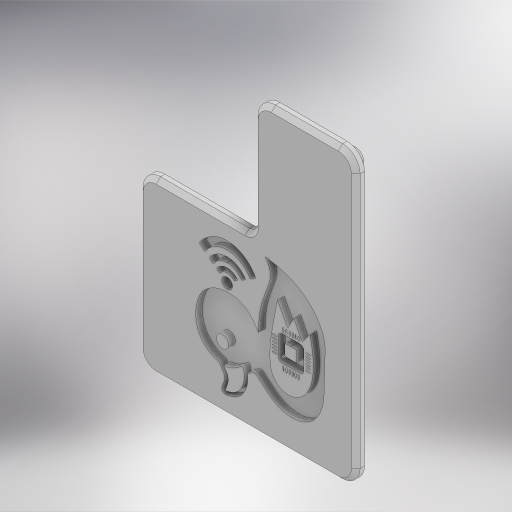
# Autodesk Inventor part: Case Top
Saved by Autodesk Inventor 2024 (Build 280153000, 153)
## iProperties
Created: 2024-10-30
Part Number: Case Top
Material: Generic
Document SubType Name: Modeling
Designer: Tejas
Mass: 8.4977 g
Surface Area: 64.1211 cm^2
Volume: 8.4977 cm^3
Density: 1 g/cm^3
Appearance: Default
Author: Tejas
Autodesk Inventor part; units mm, degrees
(part 1 of 2)
ref_plane "YZ Plane" through (0, 0, 0) normal (1, 0, 0) x (0, 1, 0)
ref_plane "XZ Plane" through (0, 0, 0) normal (0, 1, 0) x (-1, 0, 0)
ref_plane "XY Plane" through (0, 0, 0) normal (0, 0, 1) x (1, 0, 0)
sketch "Sketch1" plane through (0, 0, 0) normal (0, 0, 1) x (1, 0, 0)
  line L0 (-0.4879, 5.82) -> (-20.8921, 5.82) projected
  line L1 (-24.8921, 1.82) -> (-24.8921, -29.28) projected
  line L2 (-20.8921, -33.28) -> (20.8921, -33.28) projected
  line L3 (24.8921, -29.28) -> (24.8921, 29.28) projected
  line L4 (20.8921, 33.28) -> (5.5121, 33.28) projected
  line L5 (1.5121, 29.28) -> (1.5121, 7.82) projected
  line L6 (-22.8921, -29.28) -> (-22.8921, 1.82) projected
  line L7 (-20.8921, 3.82) -> (-0.4879, 3.82) projected
  line L8 (3.5121, 7.82) -> (3.5121, 29.28) projected
  line L9 (5.5121, 31.28) -> (20.8921, 31.28) projected
  line L10 (22.8921, 29.28) -> (22.8921, -29.28) projected
  line L11 (20.8921, -31.28) -> (-20.8921, -31.28) projected
  arc A0 (5.5121, 33.28) -> (1.5121, 29.28) centre (5.5121, 29.28) ccw projected
  arc A1 (-0.4879, 5.82) -> (1.5121, 7.82) centre (-0.4879, 7.82) ccw projected
  arc A2 (-20.8921, 5.82) -> (-24.8921, 1.82) centre (-20.8921, 1.82) ccw projected
  arc A3 (-24.8921, -29.28) -> (-20.8921, -33.28) centre (-20.8921, -29.28) ccw projected
  arc A4 (20.8921, -33.28) -> (24.8921, -29.28) centre (20.8921, -29.28) ccw projected
  arc A5 (24.8921, 29.28) -> (20.8921, 33.28) centre (20.8921, 29.28) ccw projected
  arc A6 (-0.4879, 3.82) -> (3.5121, 7.82) centre (-0.4879, 7.82) ccw projected
  arc A7 (5.5121, 31.28) -> (3.5121, 29.28) centre (5.5121, 29.28) ccw projected
  arc A8 (22.8921, 29.28) -> (20.8921, 31.28) centre (20.8921, 29.28) ccw projected
  arc A9 (20.8921, -31.28) -> (22.8921, -29.28) centre (20.8921, -29.28) ccw projected
  arc A10 (-22.8921, -29.28) -> (-20.8921, -31.28) centre (-20.8921, -29.28) ccw projected
  arc A11 (-20.8921, 3.82) -> (-22.8921, 1.82) centre (-20.8921, 1.82) ccw projected
  line L12 (22.6921, -29.28) -> (22.6921, 29.28)
  arc A12 (22.6921, 29.28) -> (20.8921, 31.08) centre (20.8921, 29.28) ccw
  line L13 (20.8921, 31.08) -> (5.5121, 31.08)
  arc A13 (5.5121, 31.08) -> (3.7121, 29.28) centre (5.5121, 29.28) ccw
  line L14 (3.7121, 29.28) -> (3.7121, 7.82)
  arc A14 (-0.4879, 3.62) -> (3.7121, 7.82) centre (-0.4879, 7.82) ccw
  line L15 (-0.4879, 3.62) -> (-20.8921, 3.62)
  arc A15 (-20.8921, 3.62) -> (-22.6921, 1.82) centre (-20.8921, 1.82) ccw
  line L16 (-22.6921, 1.82) -> (-22.6921, -29.28)
  arc A16 (-22.6921, -29.28) -> (-20.8921, -31.08) centre (-20.8921, -29.28) ccw
  line L17 (-20.8921, -31.08) -> (20.8921, -31.08)
  arc A17 (20.8921, -31.08) -> (22.6921, -29.28) centre (20.8921, -29.28) ccw
  point P0 (0, 0)
  dimension "d8" = 0.2
  constraints: 12 end point, 12 point on circle, 6 centre point, 11 other
  measures "d8" distance between parallel lines of L10 L12
extrude "Extrusion1" add sketch "Sketch1" against normal blind 2 contours A17 L17 A16 L16 A15 L15 A14 L14 A13 L13 A12 L12
sketch "Sketch2" plane through (0, 0, 0) normal (0, 0, 1) x (1, 0, 0)
  line L0 (-0.4879, 5.82) -> (-20.8921, 5.82) projected
  line L1 (-24.8921, 1.82) -> (-24.8921, -29.28) projected
  line L2 (-20.8921, -33.28) -> (20.8921, -33.28) projected
  line L3 (24.8921, -29.28) -> (24.8921, 29.28) projected
  line L4 (20.8921, 33.28) -> (5.5121, 33.28) projected
  line L5 (1.5121, 29.28) -> (1.5121, 7.82) projected
  line L6 (-22.8921, -29.28) -> (-22.8921, 1.82) projected
  line L7 (-20.8921, 3.82) -> (-0.4879, 3.82) projected
  line L8 (3.5121, 7.82) -> (3.5121, 29.28) projected
  line L9 (5.5121, 31.28) -> (20.8921, 31.28) projected
  line L10 (22.8921, 29.28) -> (22.8921, -29.28) projected
  line L11 (20.8921, -31.28) -> (-20.8921, -31.28) projected
  arc A0 (5.5121, 33.28) -> (1.5121, 29.28) centre (5.5121, 29.28) ccw projected
  arc A1 (-0.4879, 5.82) -> (1.5121, 7.82) centre (-0.4879, 7.82) ccw projected
  arc A2 (-20.8921, 5.82) -> (-24.8921, 1.82) centre (-20.8921, 1.82) ccw projected
  arc A3 (-24.8921, -29.28) -> (-20.8921, -33.28) centre (-20.8921, -29.28) ccw projected
  arc A4 (20.8921, -33.28) -> (24.8921, -29.28) centre (20.8921, -29.28) ccw projected
  arc A5 (24.8921, 29.28) -> (20.8921, 33.28) centre (20.8921, 29.28) ccw projected
  arc A6 (-0.4879, 3.82) -> (3.5121, 7.82) centre (-0.4879, 7.82) ccw projected
  arc A7 (5.5121, 31.28) -> (3.5121, 29.28) centre (5.5121, 29.28) ccw projected
  arc A8 (22.8921, 29.28) -> (20.8921, 31.28) centre (20.8921, 29.28) ccw projected
  arc A9 (20.8921, -31.28) -> (22.8921, -29.28) centre (20.8921, -29.28) ccw projected
  arc A10 (-22.8921, -29.28) -> (-20.8921, -31.28) centre (-20.8921, -29.28) ccw projected
  arc A11 (-20.8921, 3.82) -> (-22.8921, 1.82) centre (-20.8921, 1.82) ccw projected
  point P0 (0, 0)
extrude "Extrusion2" add sketch "Sketch2" along normal blind 2 contours A1 L5 A0 L4 A5 L3 A4 L2 A3 L1 A2 L0 | L6 A11 L7 A6 L8 A7 L9 A8 L10 A9 L11 A10
chamfer "Chamfer1" distance 1 angle 45 6 edges at (24.8921, 0, 2) (1.5121, 18.55, 2) (13.2021, 33.28, 2) (0, -33.28, 2) (-10.69, 5.82, 2) (-24.8921, -13.73, 2)
sketch "Sketch4" plane through (0, 0, 2) normal (0, 0, 1) x (1, 0, 0)
  spline S0 degree 3 poles (-4.7547, -28.9771) (-4.8805, -28.9733) (-5.0063, -28.9695) (-5.1321, -28.9657) (-5.8907, -28.5868) (-5.9479, -28.443) (-5.6662, -27.62) (-5.5577, -27.3029) (-5.4588, -26.9821) (-5.3379, -26.6697) (-5.0229, -25.8558) (-5.1151, -25.1226) (-5.6877, -24.4383) (-5.9033, -24.1806) (-6.0256, -23.8461) (-6.2014, -23.5532) (-6.2606, -23.4547) (-6.3372, -23.3352) (-6.4342, -23.2966) (-6.8229, -23.1422) (-7.2329, -23.0398) (-7.6166, -22.8751) (-9.6331, -22.0092) (-11.0259, -20.5743) (-11.5642, -18.4089) (-11.9734, -16.763) (-11.8527, -15.1208) (-11.3852, -13.5043) (-10.8906, -11.794) (-9.9099, -10.4354) (-8.3657, -9.5182) (-7.2061, -8.8296) (-5.9386, -8.5074) (-4.5948, -8.4534) (-3.1591, -8.3957) (-1.8032, -8.6617) (-0.5553, -9.3989) (0.7341, -10.1606) (1.5848, -11.3212) (2.3369, -12.5725) (2.4006, -12.6785) (2.4781, -12.7761) (2.5671, -12.9032) (2.5972, -12.8263) (2.6107, -12.8073) (2.6113, -12.7878) (2.6219, -12.4524) (2.6367, -12.1171) (2.6394, -11.7816) (2.6549, -9.9042) (2.9115, -8.0595) (3.4803, -6.2714) (3.8928, -4.9747) (4.3624, -3.6951) (4.8418, -2.4211) (5.558, -0.5179) (5.5086, 1.271) (4.1517, 2.8981) (4.2561, 2.8999) (4.364, 2.9203) (4.4642, 2.9007) (5.593, 2.6802) (6.7441, 2.5344) (7.8442, 2.2139) (11.5215, 1.1427) (14.5774, -0.8201) (16.5671, -4.1949) (17.399, -5.6059) (17.9137, -7.1329) (17.8745, -8.7927) (17.8045, -11.76) (17.7022, -14.7265) (17.6152, -17.6934) (17.5831, -18.7897) (17.4089, -19.8619) (17.0649, -20.9033) (16.6156, -22.2633) (15.9155, -23.4718) (14.7932, -24.3853) (12.9156, -25.9135) (10.761, -26.2581) (8.4518, -25.7287) (6.7621, -25.3413) (5.3811, -24.3687) (4.0943, -23.2515) (3.5164, -22.7497) (2.9519, -22.2318) (2.3622, -21.7443) (1.8553, -21.3253) (1.6817, -21.3258) (1.1206, -21.6528) (0.8489, -21.8111) (0.5904, -21.993) (0.3142, -22.1426) (0.1194, -22.2482) (0.0648, -22.3869) (0.078, -22.6006) (0.1026, -22.9968) (0.1327, -23.3977) (0.1005, -23.7917) (-0.0779, -25.9756) (-1.0908, -27.6067) (-3.1381, -28.4967) (-3.6499, -28.7191) (-4.2144, -28.8202) (-4.7547, -28.9771) knots 0 0 0 0 1 1 1 2 2 2 3 3 3 4 4 4 5 5 5 6 6 6 7 7 7 8 8 8 9 9 9 10 10 10 11 11 11 12 12 12 13 13 13 14 14 14 15 15 15 16 16 16 17 17 17 18 18 18 19 19 19 20 20 20 21 21 21 22 22 22 23 23 23 24 24 24 25 25 25 26 26 26 27 27 27 28 28 28 29 29 29 30 30 30 31 31 31 32 32 32 33 33 33 34 34 34 35 35 35 35
  line L0 (-4.7547, -28.9771) -> (-4.8805, -28.9733) construction
  line L1 (-4.8805, -28.9733) -> (-5.0063, -28.9695) construction
  line L2 (-5.0063, -28.9695) -> (-5.1321, -28.9657) construction
  line L3 (-5.1321, -28.9657) -> (-5.8907, -28.5868) construction
  line L4 (-5.8907, -28.5868) -> (-5.9479, -28.443) construction
  line L5 (-5.9479, -28.443) -> (-5.6662, -27.62) construction
  line L6 (-5.6662, -27.62) -> (-5.5577, -27.3029) construction
  line L7 (-5.5577, -27.3029) -> (-5.4588, -26.9821) construction
  line L8 (-5.4588, -26.9821) -> (-5.3379, -26.6697) construction
  line L9 (-5.3379, -26.6697) -> (-5.0229, -25.8558) construction
  line L10 (-5.0229, -25.8558) -> (-5.1151, -25.1226) construction
  line L11 (-5.1151, -25.1226) -> (-5.6877, -24.4383) construction
  line L12 (-5.6877, -24.4383) -> (-5.9033, -24.1806) construction
  line L13 (-5.9033, -24.1806) -> (-6.0256, -23.8461) construction
  line L14 (-6.0256, -23.8461) -> (-6.2014, -23.5532) construction
  line L15 (-6.2014, -23.5532) -> (-6.2606, -23.4547) construction
  line L16 (-6.2606, -23.4547) -> (-6.3372, -23.3352) construction
  line L17 (-6.3372, -23.3352) -> (-6.4342, -23.2966) construction
  line L18 (-6.4342, -23.2966) -> (-6.8229, -23.1422) construction
  line L19 (-6.8229, -23.1422) -> (-7.2329, -23.0398) construction
  line L20 (-7.2329, -23.0398) -> (-7.6166, -22.8751) construction
  line L21 (-7.6166, -22.8751) -> (-9.6331, -22.0092) construction
  line L22 (-9.6331, -22.0092) -> (-11.0259, -20.5743) construction
  line L23 (-11.0259, -20.5743) -> (-11.5642, -18.4089) construction
  line L24 (-11.5642, -18.4089) -> (-11.9734, -16.763) construction
  line L25 (-11.9734, -16.763) -> (-11.8527, -15.1208) construction
  line L26 (-11.8527, -15.1208) -> (-11.3852, -13.5043) construction
  line L27 (-11.3852, -13.5043) -> (-10.8906, -11.794) construction
  line L28 (-10.8906, -11.794) -> (-9.9099, -10.4354) construction
  line L29 (-9.9099, -10.4354) -> (-8.3657, -9.5182) construction
  line L30 (-8.3657, -9.5182) -> (-7.2061, -8.8296) construction
  line L31 (-7.2061, -8.8296) -> (-5.9386, -8.5074) construction
  line L32 (-5.9386, -8.5074) -> (-4.5948, -8.4534) construction
  line L33 (-4.5948, -8.4534) -> (-3.1591, -8.3957) construction
  line L34 (-3.1591, -8.3957) -> (-1.8032, -8.6617) construction
  line L35 (-1.8032, -8.6617) -> (-0.5553, -9.3989) construction
  line L36 (-0.5553, -9.3989) -> (0.7341, -10.1606) construction
  line L37 (0.7341, -10.1606) -> (1.5848, -11.3212) construction
  line L38 (1.5848, -11.3212) -> (2.3369, -12.5725) construction
  line L39 (2.3369, -12.5725) -> (2.4006, -12.6785) construction
  line L40 (2.4006, -12.6785) -> (2.4781, -12.7761) construction
  line L41 (2.4781, -12.7761) -> (2.5671, -12.9032) construction
  line L42 (2.5671, -12.9032) -> (2.5972, -12.8263) construction
  line L43 (2.5972, -12.8263) -> (2.6107, -12.8073) construction
  line L44 (2.6107, -12.8073) -> (2.6113, -12.7878) construction
  line L45 (2.6113, -12.7878) -> (2.6219, -12.4524) construction
  line L46 (2.6219, -12.4524) -> (2.6367, -12.1171) construction
  line L47 (2.6367, -12.1171) -> (2.6394, -11.7816) construction
  line L48 (2.6394, -11.7816) -> (2.6549, -9.9042) construction
  line L49 (2.6549, -9.9042) -> (2.9115, -8.0595) construction
  line L50 (2.9115, -8.0595) -> (3.4803, -6.2714) construction
  line L51 (3.4803, -6.2714) -> (3.8928, -4.9747) construction
  line L52 (3.8928, -4.9747) -> (4.3624, -3.6951) construction
  line L53 (4.3624, -3.6951) -> (4.8418, -2.4211) construction
  line L54 (4.8418, -2.4211) -> (5.558, -0.5179) construction
  line L55 (5.558, -0.5179) -> (5.5086, 1.271) construction
  line L56 (5.5086, 1.271) -> (4.1517, 2.8981) construction
  line L57 (4.1517, 2.8981) -> (4.2561, 2.8999) construction
  line L58 (4.2561, 2.8999) -> (4.364, 2.9203) construction
  line L59 (4.364, 2.9203) -> (4.4642, 2.9007) construction
  line L60 (4.4642, 2.9007) -> (5.593, 2.6802) construction
  line L61 (5.593, 2.6802) -> (6.7441, 2.5344) construction
  line L62 (6.7441, 2.5344) -> (7.8442, 2.2139) construction
  line L63 (7.8442, 2.2139) -> (11.5215, 1.1427) construction
  line L64 (11.5215, 1.1427) -> (14.5774, -0.8201) construction
  line L65 (14.5774, -0.8201) -> (16.5671, -4.1949) construction
  line L66 (16.5671, -4.1949) -> (17.399, -5.6059) construction
  line L67 (17.399, -5.6059) -> (17.9137, -7.1329) construction
  line L68 (17.9137, -7.1329) -> (17.8745, -8.7927) construction
  line L69 (17.8745, -8.7927) -> (17.8045, -11.76) construction
  line L70 (17.8045, -11.76) -> (17.7022, -14.7265) construction
  line L71 (17.7022, -14.7265) -> (17.6152, -17.6934) construction
  line L72 (17.6152, -17.6934) -> (17.5831, -18.7897) construction
  line L73 (17.5831, -18.7897) -> (17.4089, -19.8619) construction
  line L74 (17.4089, -19.8619) -> (17.0649, -20.9033) construction
  line L75 (17.0649, -20.9033) -> (16.6156, -22.2633) construction
  line L76 (16.6156, -22.2633) -> (15.9155, -23.4718) construction
  line L77 (15.9155, -23.4718) -> (14.7932, -24.3853) construction
  line L78 (14.7932, -24.3853) -> (12.9156, -25.9135) construction
  line L79 (12.9156, -25.9135) -> (10.761, -26.2581) construction
  line L80 (10.761, -26.2581) -> (8.4518, -25.7287) construction
  line L81 (8.4518, -25.7287) -> (6.7621, -25.3413) construction
  line L82 (6.7621, -25.3413) -> (5.3811, -24.3687) construction
  line L83 (5.3811, -24.3687) -> (4.0943, -23.2515) construction
  line L84 (4.0943, -23.2515) -> (3.5164, -22.7497) construction
  line L85 (3.5164, -22.7497) -> (2.9519, -22.2318) construction
  line L86 (2.9519, -22.2318) -> (2.3622, -21.7443) construction
  line L87 (2.3622, -21.7443) -> (1.8553, -21.3253) construction
  line L88 (1.8553, -21.3253) -> (1.6817, -21.3258) construction
  line L89 (1.6817, -21.3258) -> (1.1206, -21.6528) construction
  line L90 (1.1206, -21.6528) -> (0.8489, -21.8111) construction
  line L91 (0.8489, -21.8111) -> (0.5904, -21.993) construction
  line L92 (0.5904, -21.993) -> (0.3142, -22.1426) construction
  line L93 (0.3142, -22.1426) -> (0.1194, -22.2482) construction
  line L94 (0.1194, -22.2482) -> (0.0648, -22.3869) construction
  line L95 (0.0648, -22.3869) -> (0.078, -22.6006) construction
  line L96 (0.078, -22.6006) -> (0.1026, -22.9968) construction
  line L97 (0.1026, -22.9968) -> (0.1327, -23.3977) construction
  line L98 (0.1327, -23.3977) -> (0.1005, -23.7917) construction
  line L99 (0.1005, -23.7917) -> (-0.0779, -25.9756) construction
  line L100 (-0.0779, -25.9756) -> (-1.0908, -27.6067) construction
  line L101 (-1.0908, -27.6067) -> (-3.1381, -28.4967) construction
  line L102 (-3.1381, -28.4967) -> (-3.6499, -28.7191) construction
  line L103 (-3.6499, -28.7191) -> (-4.2144, -28.8202) construction
  line L104 (-4.2144, -28.8202) -> (-4.7547, -28.9771) construction
  spline S1 degree 3 poles (9.2856, -8.6579) (8.505, -7.185) (7.7646, -5.7881) (6.9636, -4.2766) (6.8805, -4.5615) (6.8204, -4.716) (6.7909, -4.8762) (6.3945, -7.025) (5.9735, -9.1697) (5.6179, -11.3252) (5.3014, -13.2442) (5.0982, -15.1784) (5.227, -17.1303) (5.2926, -18.1244) (5.4253, -19.0989) (6.0236, -19.9476) (6.7432, -20.9684) (7.6383, -21.725) (8.9273, -21.86) (10.737, -22.0495) (12.1366, -21.2461) (13.261, -19.925) (14.5002, -18.4692) (14.9367, -16.693) (15.102, -14.8381) (15.2756, -12.8887) (15.0995, -10.9567) (14.7416, -9.039) (14.6495, -8.5456) (14.5211, -8.059) (14.3809, -7.4445) (13.754, -8.2869) (13.2112, -9.0163) (12.6262, -9.8024) (12.2927, -9.142) (11.9917, -8.545) (11.6898, -7.9486) (11.3848, -7.3461) (11.0787, -6.7441) (10.7268, -6.0506) (10.2252, -6.9581) (9.7787, -7.7658) (9.2856, -8.6579) knots 0 0 0 0 1 1 1 2 2 2 3 3 3 4 4 4 5 5 5 6 6 6 7 7 7 8 8 8 9 9 9 10 10 10 11 11 11 12 12 12 13 13 13 14 14 14 14
  line L105 (9.2856, -8.6579) -> (8.505, -7.185) construction
  line L106 (8.505, -7.185) -> (7.7646, -5.7881) construction
  line L107 (7.7646, -5.7881) -> (6.9636, -4.2766) construction
  line L108 (6.9636, -4.2766) -> (6.8805, -4.5615) construction
  line L109 (6.8805, -4.5615) -> (6.8204, -4.716) construction
  line L110 (6.8204, -4.716) -> (6.7909, -4.8762) construction
  line L111 (6.7909, -4.8762) -> (6.3945, -7.025) construction
  line L112 (6.3945, -7.025) -> (5.9735, -9.1697) construction
  line L113 (5.9735, -9.1697) -> (5.6179, -11.3252) construction
  line L114 (5.6179, -11.3252) -> (5.3014, -13.2442) construction
  line L115 (5.3014, -13.2442) -> (5.0982, -15.1784) construction
  line L116 (5.0982, -15.1784) -> (5.227, -17.1303) construction
  line L117 (5.227, -17.1303) -> (5.2926, -18.1244) construction
  line L118 (5.2926, -18.1244) -> (5.4253, -19.0989) construction
  line L119 (5.4253, -19.0989) -> (6.0236, -19.9476) construction
  line L120 (6.0236, -19.9476) -> (6.7432, -20.9684) construction
  line L121 (6.7432, -20.9684) -> (7.6383, -21.725) construction
  line L122 (7.6383, -21.725) -> (8.9273, -21.86) construction
  line L123 (8.9273, -21.86) -> (10.737, -22.0495) construction
  line L124 (10.737, -22.0495) -> (12.1366, -21.2461) construction
  line L125 (12.1366, -21.2461) -> (13.261, -19.925) construction
  line L126 (13.261, -19.925) -> (14.5002, -18.4692) construction
  line L127 (14.5002, -18.4692) -> (14.9367, -16.693) construction
  line L128 (14.9367, -16.693) -> (15.102, -14.8381) construction
  line L129 (15.102, -14.8381) -> (15.2756, -12.8887) construction
  line L130 (15.2756, -12.8887) -> (15.0995, -10.9567) construction
  line L131 (15.0995, -10.9567) -> (14.7416, -9.039) construction
  line L132 (14.7416, -9.039) -> (14.6495, -8.5456) construction
  line L133 (14.6495, -8.5456) -> (14.5211, -8.059) construction
  line L134 (14.5211, -8.059) -> (14.3809, -7.4445) construction
  line L135 (14.3809, -7.4445) -> (13.754, -8.2869) construction
  line L136 (13.754, -8.2869) -> (13.2112, -9.0163) construction
  line L137 (13.2112, -9.0163) -> (12.6262, -9.8024) construction
  line L138 (12.6262, -9.8024) -> (12.2927, -9.142) construction
  line L139 (12.2927, -9.142) -> (11.9917, -8.545) construction
  line L140 (11.9917, -8.545) -> (11.6898, -7.9486) construction
  line L141 (11.6898, -7.9486) -> (11.3848, -7.3461) construction
  line L142 (11.3848, -7.3461) -> (11.0787, -6.7441) construction
  line L143 (11.0787, -6.7441) -> (10.7268, -6.0506) construction
  line L144 (10.7268, -6.0506) -> (10.2252, -6.9581) construction
  line L145 (10.2252, -6.9581) -> (9.7787, -7.7658) construction
  line L146 (9.7787, -7.7658) -> (9.2856, -8.6579) construction
  spline S2 degree 3 poles (-5.0153, -28.1685) (-4.8274, -28.1602) (-4.6842, -28.1705) (-4.5476, -28.1454) (-2.5666, -27.7822) (-1.1512, -26.3731) (-0.7618, -24.3571) (-0.5991, -23.5147) (-0.5871, -22.6719) (-0.8937, -21.8491) (-0.9953, -21.5764) (-1.1301, -21.4703) (-1.3993, -21.6813) (-1.6048, -21.8423) (-1.8351, -21.9712) (-2.0505, -22.12) (-2.978, -22.7607) (-3.9132, -23.3735) (-5.1093, -23.3633) (-5.3384, -23.3613) (-5.4382, -23.4962) (-5.2645, -23.7144) (-5.2059, -23.7881) (-5.1567, -23.8696) (-5.0954, -23.9408) (-4.3518, -24.8046) (-4.1806, -25.7695) (-4.5686, -26.8406) (-4.7209, -27.2611) (-4.8545, -27.6885) (-5.0153, -28.1685) knots 0 0 0 0 1 1 1 2 2 2 3 3 3 4 4 4 5 5 5 6 6 6 7 7 7 8 8 8 9 9 9 10 10 10 10
  line L147 (-5.0153, -28.1685) -> (-4.8274, -28.1602) construction
  line L148 (-4.8274, -28.1602) -> (-4.6842, -28.1705) construction
  line L149 (-4.6842, -28.1705) -> (-4.5476, -28.1454) construction
  line L150 (-4.5476, -28.1454) -> (-2.5666, -27.7822) construction
  line L151 (-2.5666, -27.7822) -> (-1.1512, -26.3731) construction
  line L152 (-1.1512, -26.3731) -> (-0.7618, -24.3571) construction
  line L153 (-0.7618, -24.3571) -> (-0.5991, -23.5147) construction
  line L154 (-0.5991, -23.5147) -> (-0.5871, -22.6719) construction
  line L155 (-0.5871, -22.6719) -> (-0.8937, -21.8491) construction
  line L156 (-0.8937, -21.8491) -> (-0.9953, -21.5764) construction
  line L157 (-0.9953, -21.5764) -> (-1.1301, -21.4703) construction
  line L158 (-1.1301, -21.4703) -> (-1.3993, -21.6813) construction
  line L159 (-1.3993, -21.6813) -> (-1.6048, -21.8423) construction
  line L160 (-1.6048, -21.8423) -> (-1.8351, -21.9712) construction
  line L161 (-1.8351, -21.9712) -> (-2.0505, -22.12) construction
  line L162 (-2.0505, -22.12) -> (-2.978, -22.7607) construction
  line L163 (-2.978, -22.7607) -> (-3.9132, -23.3735) construction
  line L164 (-3.9132, -23.3735) -> (-5.1093, -23.3633) construction
  line L165 (-5.1093, -23.3633) -> (-5.3384, -23.3613) construction
  line L166 (-5.3384, -23.3613) -> (-5.4382, -23.4962) construction
  line L167 (-5.4382, -23.4962) -> (-5.2645, -23.7144) construction
  line L168 (-5.2645, -23.7144) -> (-5.2059, -23.7881) construction
  line L169 (-5.2059, -23.7881) -> (-5.1567, -23.8696) construction
  line L170 (-5.1567, -23.8696) -> (-5.0954, -23.9408) construction
  line L171 (-5.0954, -23.9408) -> (-4.3518, -24.8046) construction
  line L172 (-4.3518, -24.8046) -> (-4.1806, -25.7695) construction
  line L173 (-4.1806, -25.7695) -> (-4.5686, -26.8406) construction
  line L174 (-4.5686, -26.8406) -> (-4.7209, -27.2611) construction
  line L175 (-4.7209, -27.2611) -> (-4.8545, -27.6885) construction
  line L176 (-4.8545, -27.6885) -> (-5.0153, -28.1685) construction
  spline S3 degree 3 poles (-7.051, -18.7799) (-7.0738, -19.5635) (-6.4782, -20.1949) (-5.6968, -20.2154) (-4.9245, -20.2357) (-4.2739, -19.6233) (-4.2516, -18.8549) (-4.2296, -18.0955) (-4.8598, -17.4325) (-5.6215, -17.4139) (-6.4023, -17.3948) (-7.028, -17.9928) (-7.051, -18.7799) knots 0 0 0 0 1 1 1 2 2 2 3 3 3 4 4 4 4
  line L177 (-7.051, -18.7799) -> (-7.0738, -19.5635) construction
  line L178 (-7.0738, -19.5635) -> (-6.4782, -20.1949) construction
  line L179 (-6.4782, -20.1949) -> (-5.6968, -20.2154) construction
  line L180 (-5.6968, -20.2154) -> (-4.9245, -20.2357) construction
  line L181 (-4.9245, -20.2357) -> (-4.2739, -19.6233) construction
  line L182 (-4.2739, -19.6233) -> (-4.2516, -18.8549) construction
  line L183 (-4.2516, -18.8549) -> (-4.2296, -18.0955) construction
  line L184 (-4.2296, -18.0955) -> (-4.8598, -17.4325) construction
  line L185 (-4.8598, -17.4325) -> (-5.6215, -17.4139) construction
  line L186 (-5.6215, -17.4139) -> (-6.4023, -17.3948) construction
  line L187 (-6.4023, -17.3948) -> (-7.028, -17.9928) construction
  line L188 (-7.028, -17.9928) -> (-7.051, -18.7799) construction
  spline S4 degree 3 poles (8.9341, -17.736) (8.9109, -17.6399) (8.8729, -17.5445) (8.8676, -17.4473) (8.857, -17.2539) (8.8547, -17.0587) (8.8704, -16.8659) (8.8751, -16.8074) (8.9423, -16.7183) (8.9946, -16.707) (9.0959, -16.6851) (9.1302, -16.7745) (9.1308, -16.8654) (9.1323, -17.0958) (9.1361, -17.3263) (9.1283, -17.5565) (9.1262, -17.617) (9.085, -17.6762) (9.0618, -17.736) (9.0192, -17.736) (8.9767, -17.736) (8.9341, -17.736) knots 0 0 0 0 1 1 1 2 2 2 3 3 3 4 4 4 5 5 5 6 6 6 7 7 7 7
  line L189 (8.9341, -17.736) -> (8.9109, -17.6399) construction
  line L190 (8.9109, -17.6399) -> (8.8729, -17.5445) construction
  line L191 (8.8729, -17.5445) -> (8.8676, -17.4473) construction
  line L192 (8.8676, -17.4473) -> (8.857, -17.2539) construction
  line L193 (8.857, -17.2539) -> (8.8547, -17.0587) construction
  line L194 (8.8547, -17.0587) -> (8.8704, -16.8659) construction
  line L195 (8.8704, -16.8659) -> (8.8751, -16.8074) construction
  line L196 (8.8751, -16.8074) -> (8.9423, -16.7183) construction
  line L197 (8.9423, -16.7183) -> (8.9946, -16.707) construction
  line L198 (8.9946, -16.707) -> (9.0959, -16.6851) construction
  line L199 (9.0959, -16.6851) -> (9.1302, -16.7745) construction
  line L200 (9.1302, -16.7745) -> (9.1308, -16.8654) construction
  line L201 (9.1308, -16.8654) -> (9.1323, -17.0958) construction
  line L202 (9.1323, -17.0958) -> (9.1361, -17.3263) construction
  line L203 (9.1361, -17.3263) -> (9.1283, -17.5565) construction
  line L204 (9.1283, -17.5565) -> (9.1262, -17.617) construction
  line L205 (9.1262, -17.617) -> (9.085, -17.6762) construction
  line L206 (9.085, -17.6762) -> (9.0618, -17.736) construction
  line L207 (9.0618, -17.736) -> (9.0192, -17.736) construction
  line L208 (9.0192, -17.736) -> (8.9767, -17.736) construction
  line L209 (8.9767, -17.736) -> (8.9341, -17.736) construction
  spline S5 degree 3 poles (5.7963, -14.2881) (5.8955, -14.2649) (5.9939, -14.2272) (6.0942, -14.2215) (6.2846, -14.2108) (6.4769, -14.2086) (6.6667, -14.2243) (6.7252, -14.2291) (6.7778, -14.3037) (6.8331, -14.3463) (6.781, -14.3927) (6.7311, -14.4758) (6.6763, -14.4791) (6.4377, -14.4938) (6.1974, -14.4894) (5.9581, -14.482) (5.9035, -14.4803) (5.8502, -14.4389) (5.7963, -14.4158) (5.7963, -14.3732) (5.7963, -14.3306) (5.7963, -14.2881) knots 0 0 0 0 1 1 1 2 2 2 3 3 3 4 4 4 5 5 5 6 6 6 7 7 7 7
  line L210 (5.7963, -14.2881) -> (5.8955, -14.2649) construction
  line L211 (5.8955, -14.2649) -> (5.9939, -14.2272) construction
  line L212 (5.9939, -14.2272) -> (6.0942, -14.2215) construction
  line L213 (6.0942, -14.2215) -> (6.2846, -14.2108) construction
  line L214 (6.2846, -14.2108) -> (6.4769, -14.2086) construction
  line L215 (6.4769, -14.2086) -> (6.6667, -14.2243) construction
  line L216 (6.6667, -14.2243) -> (6.7252, -14.2291) construction
  line L217 (6.7252, -14.2291) -> (6.7778, -14.3037) construction
  line L218 (6.7778, -14.3037) -> (6.8331, -14.3463) construction
  line L219 (6.8331, -14.3463) -> (6.781, -14.3927) construction
  line L220 (6.781, -14.3927) -> (6.7311, -14.4758) construction
  line L221 (6.7311, -14.4758) -> (6.6763, -14.4791) construction
  line L222 (6.6763, -14.4791) -> (6.4377, -14.4938) construction
  line L223 (6.4377, -14.4938) -> (6.1974, -14.4894) construction
  line L224 (6.1974, -14.4894) -> (5.9581, -14.482) construction
  line L225 (5.9581, -14.482) -> (5.9035, -14.4803) construction
  line L226 (5.9035, -14.4803) -> (5.8502, -14.4389) construction
  line L227 (5.8502, -14.4389) -> (5.7963, -14.4158) construction
  line L228 (5.7963, -14.4158) -> (5.7963, -14.3732) construction
  line L229 (5.7963, -14.3732) -> (5.7963, -14.3306) construction
  line L230 (5.7963, -14.3306) -> (5.7963, -14.2881) construction
  spline S6 degree 3 poles (5.7963, -11.5151) (5.9231, -11.4928) (6.0491, -11.4594) (6.1768, -11.4508) (6.3428, -11.4396) (6.5113, -11.4365) (6.6761, -11.4545) (6.7326, -11.4607) (6.7811, -11.541) (6.8332, -11.5874) (6.7805, -11.6291) (6.7296, -11.7038) (6.6748, -11.7069) (6.436, -11.7202) (6.196, -11.7169) (5.9567, -11.7096) (5.9026, -11.7079) (5.8497, -11.6661) (5.7963, -11.6428) (5.7963, -11.6003) (5.7963, -11.5577) (5.7963, -11.5151) knots 0 0 0 0 1 1 1 2 2 2 3 3 3 4 4 4 5 5 5 6 6 6 7 7 7 7
  line L231 (5.7963, -11.5151) -> (5.9231, -11.4928) construction
  line L232 (5.9231, -11.4928) -> (6.0491, -11.4594) construction
  line L233 (6.0491, -11.4594) -> (6.1768, -11.4508) construction
  line L234 (6.1768, -11.4508) -> (6.3428, -11.4396) construction
  line L235 (6.3428, -11.4396) -> (6.5113, -11.4365) construction
  line L236 (6.5113, -11.4365) -> (6.6761, -11.4545) construction
  line L237 (6.6761, -11.4545) -> (6.7326, -11.4607) construction
  line L238 (6.7326, -11.4607) -> (6.7811, -11.541) construction
  line L239 (6.7811, -11.541) -> (6.8332, -11.5874) construction
  line L240 (6.8332, -11.5874) -> (6.7805, -11.6291) construction
  line L241 (6.7805, -11.6291) -> (6.7296, -11.7038) construction
  line L242 (6.7296, -11.7038) -> (6.6748, -11.7069) construction
  line L243 (6.6748, -11.7069) -> (6.436, -11.7202) construction
  line L244 (6.436, -11.7202) -> (6.196, -11.7169) construction
  line L245 (6.196, -11.7169) -> (5.9567, -11.7096) construction
  line L246 (5.9567, -11.7096) -> (5.9026, -11.7079) construction
  line L247 (5.9026, -11.7079) -> (5.8497, -11.6661) construction
  line L248 (5.8497, -11.6661) -> (5.7963, -11.6428) construction
  line L249 (5.7963, -11.6428) -> (5.7963, -11.6003) construction
  line L250 (5.7963, -11.6003) -> (5.7963, -11.5577) construction
  line L251 (5.7963, -11.5577) -> (5.7963, -11.5151) construction
  spline S7 degree 3 poles (11.6888, -17.736) (11.6717, -17.4297) (11.6503, -17.1235) (11.6431, -16.817) (11.6422, -16.7787) (11.717, -16.7073) (11.7563, -16.7076) (11.801, -16.7079) (11.8824, -16.7699) (11.8839, -16.8078) (11.8949, -17.0771) (11.8918, -17.3472) (11.8869, -17.6169) (11.8862, -17.6569) (11.853, -17.6963) (11.8348, -17.736) (11.7861, -17.736) (11.7375, -17.736) (11.6888, -17.736) knots 0 0 0 0 1 1 1 2 2 2 3 3 3 4 4 4 5 5 5 6 6 6 6
  line L252 (11.6888, -17.736) -> (11.6717, -17.4297) construction
  line L253 (11.6717, -17.4297) -> (11.6503, -17.1235) construction
  line L254 (11.6503, -17.1235) -> (11.6431, -16.817) construction
  line L255 (11.6431, -16.817) -> (11.6422, -16.7787) construction
  line L256 (11.6422, -16.7787) -> (11.717, -16.7073) construction
  line L257 (11.717, -16.7073) -> (11.7563, -16.7076) construction
  line L258 (11.7563, -16.7076) -> (11.801, -16.7079) construction
  line L259 (11.801, -16.7079) -> (11.8824, -16.7699) construction
  line L260 (11.8824, -16.7699) -> (11.8839, -16.8078) construction
  line L261 (11.8839, -16.8078) -> (11.8949, -17.0771) construction
  line L262 (11.8949, -17.0771) -> (11.8918, -17.3472) construction
  line L263 (11.8918, -17.3472) -> (11.8869, -17.6169) construction
  line L264 (11.8869, -17.6169) -> (11.8862, -17.6569) construction
  line L265 (11.8862, -17.6569) -> (11.853, -17.6963) construction
  line L266 (11.853, -17.6963) -> (11.8348, -17.736) construction
  line L267 (11.8348, -17.736) -> (11.7861, -17.736) construction
  line L268 (11.7861, -17.736) -> (11.7375, -17.736) construction
  line L269 (11.7375, -17.736) -> (11.6888, -17.736) construction
  spline S8 degree 3 poles (5.7963, -12.9381) (5.8836, -12.9148) (5.9702, -12.8759) (6.0585, -12.8715) (6.261, -12.8615) (6.465, -12.8592) (6.6668, -12.8743) (6.725, -12.8787) (6.8139, -12.9452) (6.8255, -12.9972) (6.8482, -13.0996) (6.7571, -13.1329) (6.6677, -13.1338) (6.4375, -13.1361) (6.2071, -13.1394) (5.9771, -13.1315) (5.9162, -13.1295) (5.8565, -13.0888) (5.7963, -13.0658) (5.7963, -13.0232) (5.7963, -12.9807) (5.7963, -12.9381) knots 0 0 0 0 1 1 1 2 2 2 3 3 3 4 4 4 5 5 5 6 6 6 7 7 7 7
  line L270 (5.7963, -12.9381) -> (5.8836, -12.9148) construction
  line L271 (5.8836, -12.9148) -> (5.9702, -12.8759) construction
  line L272 (5.9702, -12.8759) -> (6.0585, -12.8715) construction
  line L273 (6.0585, -12.8715) -> (6.261, -12.8615) construction
  line L274 (6.261, -12.8615) -> (6.465, -12.8592) construction
  line L275 (6.465, -12.8592) -> (6.6668, -12.8743) construction
  line L276 (6.6668, -12.8743) -> (6.725, -12.8787) construction
  line L277 (6.725, -12.8787) -> (6.8139, -12.9452) construction
  line L278 (6.8139, -12.9452) -> (6.8255, -12.9972) construction
  line L279 (6.8255, -12.9972) -> (6.8482, -13.0996) construction
  line L280 (6.8482, -13.0996) -> (6.7571, -13.1329) construction
  line L281 (6.7571, -13.1329) -> (6.6677, -13.1338) construction
  line L282 (6.6677, -13.1338) -> (6.4375, -13.1361) construction
  line L283 (6.4375, -13.1361) -> (6.2071, -13.1394) construction
  line L284 (6.2071, -13.1394) -> (5.9771, -13.1315) construction
  line L285 (5.9771, -13.1315) -> (5.9162, -13.1295) construction
  line L286 (5.9162, -13.1295) -> (5.8565, -13.0888) construction
  line L287 (5.8565, -13.0888) -> (5.7963, -13.0658) construction
  line L288 (5.7963, -13.0658) -> (5.7963, -13.0232) construction
  line L289 (5.7963, -13.0232) -> (5.7963, -12.9807) construction
  line L290 (5.7963, -12.9807) -> (5.7963, -12.9381) construction
  spline S9 degree 3 poles (10.9956, -17.736) (10.9742, -17.5908) (10.9427, -17.4462) (10.9343, -17.3002) (10.925, -17.1376) (10.9285, -16.973) (10.9455, -16.8112) (10.9498, -16.77) (11.0284, -16.7055) (11.0696, -16.7079) (11.1128, -16.7104) (11.1857, -16.7791) (11.1875, -16.8213) (11.1986, -17.0813) (11.1956, -17.342) (11.1909, -17.6024) (11.1901, -17.6472) (11.1587, -17.6915) (11.1415, -17.736) (11.0929, -17.736) (11.0442, -17.736) (10.9956, -17.736) knots 0 0 0 0 1 1 1 2 2 2 3 3 3 4 4 4 5 5 5 6 6 6 7 7 7 7
  line L291 (10.9956, -17.736) -> (10.9742, -17.5908) construction
  line L292 (10.9742, -17.5908) -> (10.9427, -17.4462) construction
  line L293 (10.9427, -17.4462) -> (10.9343, -17.3002) construction
  line L294 (10.9343, -17.3002) -> (10.925, -17.1376) construction
  line L295 (10.925, -17.1376) -> (10.9285, -16.973) construction
  line L296 (10.9285, -16.973) -> (10.9455, -16.8112) construction
  line L297 (10.9455, -16.8112) -> (10.9498, -16.77) construction
  line L298 (10.9498, -16.77) -> (11.0284, -16.7055) construction
  line L299 (11.0284, -16.7055) -> (11.0696, -16.7079) construction
  line L300 (11.0696, -16.7079) -> (11.1128, -16.7104) construction
  line L301 (11.1128, -16.7104) -> (11.1857, -16.7791) construction
  line L302 (11.1857, -16.7791) -> (11.1875, -16.8213) construction
  line L303 (11.1875, -16.8213) -> (11.1986, -17.0813) construction
  line L304 (11.1986, -17.0813) -> (11.1956, -17.342) construction
  line L305 (11.1956, -17.342) -> (11.1909, -17.6024) construction
  line L306 (11.1909, -17.6024) -> (11.1901, -17.6472) construction
  line L307 (11.1901, -17.6472) -> (11.1587, -17.6915) construction
  line L308 (11.1587, -17.6915) -> (11.1415, -17.736) construction
  line L309 (11.1415, -17.736) -> (11.0929, -17.736) construction
  line L310 (11.0929, -17.736) -> (11.0442, -17.736) construction
  line L311 (11.0442, -17.736) -> (10.9956, -17.736) construction
  spline S10 degree 3 poles (9.6456, -17.736) (9.624, -17.609) (9.5903, -17.4827) (9.5836, -17.3549) (9.5742, -17.177) (9.5757, -16.9971) (9.5934, -16.8202) (9.5978, -16.7759) (9.6818, -16.7396) (9.7292, -16.6997) (9.7672, -16.7464) (9.8358, -16.7917) (9.838, -16.84) (9.8492, -17.0878) (9.8472, -17.3365) (9.8402, -17.5847) (9.8388, -17.6357) (9.7966, -17.6856) (9.7733, -17.736) (9.7307, -17.736) (9.6881, -17.736) (9.6456, -17.736) knots 0 0 0 0 1 1 1 2 2 2 3 3 3 4 4 4 5 5 5 6 6 6 7 7 7 7
  line L312 (9.6456, -17.736) -> (9.624, -17.609) construction
  line L313 (9.624, -17.609) -> (9.5903, -17.4827) construction
  line L314 (9.5903, -17.4827) -> (9.5836, -17.3549) construction
  line L315 (9.5836, -17.3549) -> (9.5742, -17.177) construction
  line L316 (9.5742, -17.177) -> (9.5757, -16.9971) construction
  line L317 (9.5757, -16.9971) -> (9.5934, -16.8202) construction
  line L318 (9.5934, -16.8202) -> (9.5978, -16.7759) construction
  line L319 (9.5978, -16.7759) -> (9.6818, -16.7396) construction
  line L320 (9.6818, -16.7396) -> (9.7292, -16.6997) construction
  line L321 (9.7292, -16.6997) -> (9.7672, -16.7464) construction
  line L322 (9.7672, -16.7464) -> (9.8358, -16.7917) construction
  line L323 (9.8358, -16.7917) -> (9.838, -16.84) construction
  line L324 (9.838, -16.84) -> (9.8492, -17.0878) construction
  line L325 (9.8492, -17.0878) -> (9.8472, -17.3365) construction
  line L326 (9.8472, -17.3365) -> (9.8402, -17.5847) construction
  line L327 (9.8402, -17.5847) -> (9.8388, -17.6357) construction
  line L328 (9.8388, -17.6357) -> (9.7966, -17.6856) construction
  line L329 (9.7966, -17.6856) -> (9.7733, -17.736) construction
  line L330 (9.7733, -17.736) -> (9.7307, -17.736) construction
  line L331 (9.7307, -17.736) -> (9.6881, -17.736) construction
  line L332 (9.6881, -17.736) -> (9.6456, -17.736) construction
  spline S11 degree 3 poles (14.4435, -11.6793) (14.1457, -11.6903) (13.8479, -11.7062) (13.55, -11.7067) (13.5084, -11.7067) (13.4322, -11.63) (13.4337, -11.5913) (13.4356, -11.5439) (13.5025, -11.4598) (13.5416, -11.4596) (13.8334, -11.4583) (14.1254, -11.4739) (14.4173, -11.4838) (14.426, -11.4841) (14.4348, -11.4805) (14.4435, -11.4786) (14.4435, -11.5455) (14.4435, -11.6124) (14.4435, -11.6793) knots 0 0 0 0 1 1 1 2 2 2 3 3 3 4 4 4 5 5 5 6 6 6 6
  line L333 (14.4435, -11.6793) -> (14.1457, -11.6903) construction
  line L334 (14.1457, -11.6903) -> (13.8479, -11.7062) construction
  line L335 (13.8479, -11.7062) -> (13.55, -11.7067) construction
  line L336 (13.55, -11.7067) -> (13.5084, -11.7067) construction
  line L337 (13.5084, -11.7067) -> (13.4322, -11.63) construction
  line L338 (13.4322, -11.63) -> (13.4337, -11.5913) construction
  line L339 (13.4337, -11.5913) -> (13.4356, -11.5439) construction
  line L340 (13.4356, -11.5439) -> (13.5025, -11.4598) construction
  line L341 (13.5025, -11.4598) -> (13.5416, -11.4596) construction
  line L342 (13.5416, -11.4596) -> (13.8334, -11.4583) construction
  line L343 (13.8334, -11.4583) -> (14.1254, -11.4739) construction
  line L344 (14.1254, -11.4739) -> (14.4173, -11.4838) construction
  line L345 (14.4173, -11.4838) -> (14.426, -11.4841) construction
  line L346 (14.426, -11.4841) -> (14.4348, -11.4805) construction
  line L347 (14.4348, -11.4805) -> (14.4435, -11.4786) construction
  line L348 (14.4435, -11.4786) -> (14.4435, -11.5455) construction
  line L349 (14.4435, -11.5455) -> (14.4435, -11.6124) construction
  line L350 (14.4435, -11.6124) -> (14.4435, -11.6793) construction
  spline S12 degree 3 poles (9.0983, -9.0888) (9.1093, -9.3716) (9.128, -9.6544) (9.125, -9.9371) (9.1244, -9.9945) (9.0499, -10.0891) (8.996, -10.0999) (8.8949, -10.1203) (8.8648, -10.0283) (8.8646, -9.9377) (8.8641, -9.7101) (8.8623, -9.4825) (8.866, -9.255) (8.8669, -9.1994) (8.8866, -9.1442) (8.8976, -9.0888) (8.9645, -9.0888) (9.0314, -9.0888) (9.0983, -9.0888) knots 0 0 0 0 1 1 1 2 2 2 3 3 3 4 4 4 5 5 5 6 6 6 6
  line L351 (9.0983, -9.0888) -> (9.1093, -9.3716) construction
  line L352 (9.1093, -9.3716) -> (9.128, -9.6544) construction
  line L353 (9.128, -9.6544) -> (9.125, -9.9371) construction
  line L354 (9.125, -9.9371) -> (9.1244, -9.9945) construction
  line L355 (9.1244, -9.9945) -> (9.0499, -10.0891) construction
  line L356 (9.0499, -10.0891) -> (8.996, -10.0999) construction
  line L357 (8.996, -10.0999) -> (8.8949, -10.1203) construction
  line L358 (8.8949, -10.1203) -> (8.8648, -10.0283) construction
  line L359 (8.8648, -10.0283) -> (8.8646, -9.9377) construction
  line L360 (8.8646, -9.9377) -> (8.8641, -9.7101) construction
  line L361 (8.8641, -9.7101) -> (8.8623, -9.4825) construction
  line L362 (8.8623, -9.4825) -> (8.866, -9.255) construction
  line L363 (8.866, -9.255) -> (8.8669, -9.1994) construction
  line L364 (8.8669, -9.1994) -> (8.8866, -9.1442) construction
  line L365 (8.8866, -9.1442) -> (8.8976, -9.0888) construction
  line L366 (8.8976, -9.0888) -> (8.9645, -9.0888) construction
  line L367 (8.9645, -9.0888) -> (9.0314, -9.0888) construction
  line L368 (9.0314, -9.0888) -> (9.0983, -9.0888) construction
  spline S13 degree 3 poles (14.4435, -14.4523) (14.1578, -14.4633) (13.872, -14.4815) (13.5863, -14.479) (13.5321, -14.4785) (13.4785, -14.396) (13.4247, -14.3513) (13.4785, -14.307) (13.5301, -14.2281) (13.5864, -14.2245) (13.819, -14.2101) (14.0531, -14.2165) (14.2866, -14.22) (14.339, -14.2207) (14.3912, -14.2405) (14.4435, -14.2516) (14.4435, -14.3185) (14.4435, -14.3854) (14.4435, -14.4523) knots 0 0 0 0 1 1 1 2 2 2 3 3 3 4 4 4 5 5 5 6 6 6 6
  line L369 (14.4435, -14.4523) -> (14.1578, -14.4633) construction
  line L370 (14.1578, -14.4633) -> (13.872, -14.4815) construction
  line L371 (13.872, -14.4815) -> (13.5863, -14.479) construction
  line L372 (13.5863, -14.479) -> (13.5321, -14.4785) construction
  line L373 (13.5321, -14.4785) -> (13.4785, -14.396) construction
  line L374 (13.4785, -14.396) -> (13.4247, -14.3513) construction
  line L375 (13.4247, -14.3513) -> (13.4785, -14.307) construction
  line L376 (13.4785, -14.307) -> (13.5301, -14.2281) construction
  line L377 (13.5301, -14.2281) -> (13.5864, -14.2245) construction
  line L378 (13.5864, -14.2245) -> (13.819, -14.2101) construction
  line L379 (13.819, -14.2101) -> (14.0531, -14.2165) construction
  line L380 (14.0531, -14.2165) -> (14.2866, -14.22) construction
  line L381 (14.2866, -14.22) -> (14.339, -14.2207) construction
  line L382 (14.339, -14.2207) -> (14.3912, -14.2405) construction
  line L383 (14.3912, -14.2405) -> (14.4435, -14.2516) construction
  line L384 (14.4435, -14.2516) -> (14.4435, -14.3185) construction
  line L385 (14.4435, -14.3185) -> (14.4435, -14.3854) construction
  line L386 (14.4435, -14.3854) -> (14.4435, -14.4523) construction
  spline S14 degree 3 poles (14.4435, -13.1023) (14.164, -13.1133) (13.8846, -13.1261) (13.605, -13.1343) (13.5144, -13.1369) (13.4274, -13.1133) (13.4269, -13.0001) (13.4264, -12.8854) (13.5121, -12.8683) (13.6043, -12.8683) (13.8256, -12.8684) (14.047, -12.8661) (14.2683, -12.8699) (14.3269, -12.8709) (14.3851, -12.8905) (14.4435, -12.9016) (14.4435, -12.9685) (14.4435, -13.0354) (14.4435, -13.1023) knots 0 0 0 0 1 1 1 2 2 2 3 3 3 4 4 4 5 5 5 6 6 6 6
  line L387 (14.4435, -13.1023) -> (14.164, -13.1133) construction
  line L388 (14.164, -13.1133) -> (13.8846, -13.1261) construction
  line L389 (13.8846, -13.1261) -> (13.605, -13.1343) construction
  line L390 (13.605, -13.1343) -> (13.5144, -13.1369) construction
  line L391 (13.5144, -13.1369) -> (13.4274, -13.1133) construction
  line L392 (13.4274, -13.1133) -> (13.4269, -13.0001) construction
  line L393 (13.4269, -13.0001) -> (13.4264, -12.8854) construction
  line L394 (13.4264, -12.8854) -> (13.5121, -12.8683) construction
  line L395 (13.5121, -12.8683) -> (13.6043, -12.8683) construction
  line L396 (13.6043, -12.8683) -> (13.8256, -12.8684) construction
  line L397 (13.8256, -12.8684) -> (14.047, -12.8661) construction
  line L398 (14.047, -12.8661) -> (14.2683, -12.8699) construction
  line L399 (14.2683, -12.8699) -> (14.3269, -12.8709) construction
  line L400 (14.3269, -12.8709) -> (14.3851, -12.8905) construction
  line L401 (14.3851, -12.8905) -> (14.4435, -12.9016) construction
  line L402 (14.4435, -12.9016) -> (14.4435, -12.9685) construction
  line L403 (14.4435, -12.9685) -> (14.4435, -13.0354) construction
  line L404 (14.4435, -13.0354) -> (14.4435, -13.1023) construction
  spline S15 degree 3 poles (9.8098, -9.0888) (9.8208, -9.3898) (9.8362, -9.6909) (9.8373, -9.992) (9.8374, -10.0302) (9.7664, -10.0927) (9.7214, -10.0998) (9.6839, -10.1057) (9.5985, -10.0467) (9.5987, -10.0168) (9.6007, -9.7074) (9.6159, -9.3981) (9.6273, -9.0888) (9.6881, -9.0888) (9.749, -9.0888) (9.8098, -9.0888) knots 0 0 0 0 1 1 1 2 2 2 3 3 3 4 4 4 5 5 5 5
  line L405 (9.8098, -9.0888) -> (9.8208, -9.3898) construction
  line L406 (9.8208, -9.3898) -> (9.8362, -9.6909) construction
  line L407 (9.8362, -9.6909) -> (9.8373, -9.992) construction
  line L408 (9.8373, -9.992) -> (9.8374, -10.0302) construction
  line L409 (9.8374, -10.0302) -> (9.7664, -10.0927) construction
  line L410 (9.7664, -10.0927) -> (9.7214, -10.0998) construction
  line L411 (9.7214, -10.0998) -> (9.6839, -10.1057) construction
  line L412 (9.6839, -10.1057) -> (9.5985, -10.0467) construction
  line L413 (9.5985, -10.0467) -> (9.5987, -10.0168) construction
  line L414 (9.5987, -10.0168) -> (9.6007, -9.7074) construction
  line L415 (9.6007, -9.7074) -> (9.6159, -9.3981) construction
  line L416 (9.6159, -9.3981) -> (9.6273, -9.0888) construction
  line L417 (9.6273, -9.0888) -> (9.6881, -9.0888) construction
  line L418 (9.6881, -9.0888) -> (9.749, -9.0888) construction
  line L419 (9.749, -9.0888) -> (9.8098, -9.0888) construction
  spline S16 degree 3 poles (11.1598, -9.0888) (11.1708, -9.3899) (11.1863, -9.6909) (11.1874, -9.9921) (11.1876, -10.0304) (11.1162, -10.0927) (11.0709, -10.1001) (11.0338, -10.1061) (10.9486, -10.0465) (10.9488, -10.0164) (10.9508, -9.7072) (10.9659, -9.398) (10.9773, -9.0888) (11.0381, -9.0888) (11.099, -9.0888) (11.1598, -9.0888) knots 0 0 0 0 1 1 1 2 2 2 3 3 3 4 4 4 5 5 5 5
  line L420 (11.1598, -9.0888) -> (11.1708, -9.3899) construction
  line L421 (11.1708, -9.3899) -> (11.1863, -9.6909) construction
  line L422 (11.1863, -9.6909) -> (11.1874, -9.9921) construction
  line L423 (11.1874, -9.9921) -> (11.1876, -10.0304) construction
  line L424 (11.1876, -10.0304) -> (11.1162, -10.0927) construction
  line L425 (11.1162, -10.0927) -> (11.0709, -10.1001) construction
  line L426 (11.0709, -10.1001) -> (11.0338, -10.1061) construction
  line L427 (11.0338, -10.1061) -> (10.9486, -10.0465) construction
  line L428 (10.9486, -10.0465) -> (10.9488, -10.0164) construction
  line L429 (10.9488, -10.0164) -> (10.9508, -9.7072) construction
  line L430 (10.9508, -9.7072) -> (10.9659, -9.398) construction
  line L431 (10.9659, -9.398) -> (10.9773, -9.0888) construction
  line L432 (10.9773, -9.0888) -> (11.0381, -9.0888) construction
  line L433 (11.0381, -9.0888) -> (11.099, -9.0888) construction
  line L434 (11.099, -9.0888) -> (11.1598, -9.0888) construction
  spline S17 degree 3 poles (11.853, -9.0888) (11.8682, -9.2223) (11.8911, -9.3555) (11.8967, -9.4895) (11.9037, -9.653) (11.9061, -9.8181) (11.8888, -9.9802) (11.8838, -10.0267) (11.8039, -10.0652) (11.7583, -10.1074) (11.7179, -10.0598) (11.6449, -10.0138) (11.6425, -9.9642) (11.6304, -9.719) (11.6353, -9.4728) (11.6385, -9.227) (11.6391, -9.1808) (11.6594, -9.1349) (11.6706, -9.0888) (11.7314, -9.0888) (11.7922, -9.0888) (11.853, -9.0888) knots 0 0 0 0 1 1 1 2 2 2 3 3 3 4 4 4 5 5 5 6 6 6 7 7 7 7
  line L435 (11.853, -9.0888) -> (11.8682, -9.2223) construction
  line L436 (11.8682, -9.2223) -> (11.8911, -9.3555) construction
  line L437 (11.8911, -9.3555) -> (11.8967, -9.4895) construction
  line L438 (11.8967, -9.4895) -> (11.9037, -9.653) construction
  line L439 (11.9037, -9.653) -> (11.9061, -9.8181) construction
  line L440 (11.9061, -9.8181) -> (11.8888, -9.9802) construction
  line L441 (11.8888, -9.9802) -> (11.8838, -10.0267) construction
  line L442 (11.8838, -10.0267) -> (11.8039, -10.0652) construction
  line L443 (11.8039, -10.0652) -> (11.7583, -10.1074) construction
  line L444 (11.7583, -10.1074) -> (11.7179, -10.0598) construction
  line L445 (11.7179, -10.0598) -> (11.6449, -10.0138) construction
  line L446 (11.6449, -10.0138) -> (11.6425, -9.9642) construction
  line L447 (11.6425, -9.9642) -> (11.6304, -9.719) construction
  line L448 (11.6304, -9.719) -> (11.6353, -9.4728) construction
  line L449 (11.6353, -9.4728) -> (11.6385, -9.227) construction
  line L450 (11.6385, -9.227) -> (11.6391, -9.1808) construction
  line L451 (11.6391, -9.1808) -> (11.6594, -9.1349) construction
  line L452 (11.6594, -9.1349) -> (11.6706, -9.0888) construction
  line L453 (11.6706, -9.0888) -> (11.7314, -9.0888) construction
  line L454 (11.7314, -9.0888) -> (11.7922, -9.0888) construction
  line L455 (11.7922, -9.0888) -> (11.853, -9.0888) construction
  spline S18 degree 3 poles (5.7963, -14.9813) (6.1121, -14.9647) (6.4278, -14.9446) (6.7438, -14.9374) (6.7726, -14.9368) (6.8287, -15.0213) (6.826, -15.0632) (6.8233, -15.1039) (6.7623, -15.1727) (6.7249, -15.174) (6.4553, -15.1835) (6.1852, -15.1811) (5.9153, -15.1767) (5.8754, -15.176) (5.836, -15.1445) (5.7963, -15.1273) (5.7963, -15.0786) (5.7963, -15.03) (5.7963, -14.9813) knots 0 0 0 0 1 1 1 2 2 2 3 3 3 4 4 4 5 5 5 6 6 6 6
  line L456 (5.7963, -14.9813) -> (6.1121, -14.9647) construction
  line L457 (6.1121, -14.9647) -> (6.4278, -14.9446) construction
  line L458 (6.4278, -14.9446) -> (6.7438, -14.9374) construction
  line L459 (6.7438, -14.9374) -> (6.7726, -14.9368) construction
  line L460 (6.7726, -14.9368) -> (6.8287, -15.0213) construction
  line L461 (6.8287, -15.0213) -> (6.826, -15.0632) construction
  line L462 (6.826, -15.0632) -> (6.8233, -15.1039) construction
  line L463 (6.8233, -15.1039) -> (6.7623, -15.1727) construction
  line L464 (6.7623, -15.1727) -> (6.7249, -15.174) construction
  line L465 (6.7249, -15.174) -> (6.4553, -15.1835) construction
  line L466 (6.4553, -15.1835) -> (6.1852, -15.1811) construction
  line L467 (6.1852, -15.1811) -> (5.9153, -15.1767) construction
  line L468 (5.9153, -15.1767) -> (5.8754, -15.176) construction
  line L469 (5.8754, -15.176) -> (5.836, -15.1445) construction
  line L470 (5.836, -15.1445) -> (5.7963, -15.1273) construction
  line L471 (5.7963, -15.1273) -> (5.7963, -15.0786) construction
  line L472 (5.7963, -15.0786) -> (5.7963, -15.03) construction
  line L473 (5.7963, -15.03) -> (5.7963, -14.9813) construction
  spline S19 degree 3 poles (8.2226, -17.736) (8.2056, -17.4236) (8.1845, -17.1112) (8.1775, -16.7985) (8.1768, -16.7665) (8.2619, -16.7046) (8.3038, -16.7074) (8.345, -16.7101) (8.4141, -16.7763) (8.4156, -16.8167) (8.4258, -17.08) (8.4233, -17.3439) (8.4186, -17.6075) (8.4178, -17.6507) (8.386, -17.6932) (8.3686, -17.736) (8.3199, -17.736) (8.2713, -17.736) (8.2226, -17.736) knots 0 0 0 0 1 1 1 2 2 2 3 3 3 4 4 4 5 5 5 6 6 6 6
  line L474 (8.2226, -17.736) -> (8.2056, -17.4236) construction
  line L475 (8.2056, -17.4236) -> (8.1845, -17.1112) construction
  line L476 (8.1845, -17.1112) -> (8.1775, -16.7985) construction
  line L477 (8.1775, -16.7985) -> (8.1768, -16.7665) construction
  line L478 (8.1768, -16.7665) -> (8.2619, -16.7046) construction
  line L479 (8.2619, -16.7046) -> (8.3038, -16.7074) construction
  line L480 (8.3038, -16.7074) -> (8.345, -16.7101) construction
  line L481 (8.345, -16.7101) -> (8.4141, -16.7763) construction
  line L482 (8.4141, -16.7763) -> (8.4156, -16.8167) construction
  line L483 (8.4156, -16.8167) -> (8.4258, -17.08) construction
  line L484 (8.4258, -17.08) -> (8.4233, -17.3439) construction
  line L485 (8.4233, -17.3439) -> (8.4186, -17.6075) construction
  line L486 (8.4186, -17.6075) -> (8.4178, -17.6507) construction
  line L487 (8.4178, -17.6507) -> (8.386, -17.6932) construction
  line L488 (8.386, -17.6932) -> (8.3686, -17.736) construction
  line L489 (8.3686, -17.736) -> (8.3199, -17.736) construction
  line L490 (8.3199, -17.736) -> (8.2713, -17.736) construction
  line L491 (8.2713, -17.736) -> (8.2226, -17.736) construction
  spline S20 degree 3 poles (5.7963, -13.6313) (6.1088, -13.6141) (6.4212, -13.5932) (6.734, -13.5853) (6.7661, -13.5845) (6.8293, -13.6645) (6.8259, -13.7023) (6.8218, -13.747) (6.7624, -13.8212) (6.7246, -13.8227) (6.4551, -13.8332) (6.185, -13.8306) (5.9152, -13.8264) (5.8753, -13.8258) (5.8359, -13.7944) (5.7963, -13.7773) (5.7963, -13.7286) (5.7963, -13.68) (5.7963, -13.6313) knots 0 0 0 0 1 1 1 2 2 2 3 3 3 4 4 4 5 5 5 6 6 6 6
  line L492 (5.7963, -13.6313) -> (6.1088, -13.6141) construction
  line L493 (6.1088, -13.6141) -> (6.4212, -13.5932) construction
  line L494 (6.4212, -13.5932) -> (6.734, -13.5853) construction
  line L495 (6.734, -13.5853) -> (6.7661, -13.5845) construction